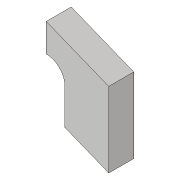
# Autodesk Inventor part: At Angle Linear Dim
Saved by Autodesk Inventor 2018.3 (Build 223284000, 284)
## iProperties
Created: 2020-03-26
Part Number: At Angle Linear Dim
Material: Generic
Document SubType Name: Modeling
Designer: MattBussey
Density: 1 g/cm^3
Appearance: Default
RuleStatus: InUse
Author: MattBussey
Autodesk Inventor part; units mm, degrees
ref_plane "YZ Plane" through (0, 0, 0) normal (1, 0, 0) x (0, 1, 0)
ref_plane "XZ Plane" through (0, 0, 0) normal (0, 1, 0) x (-1, 0, 0)
ref_plane "XY Plane" through (0, 0, 0) normal (0, 0, 1) x (1, 0, 0)
sketch "Sketch1" plane through (0, 0, 0) normal (0, 0, 1) x (1, 0, 0)
  line L0 (0, 0) -> (-63.5, 25.4)
  line L1 (-63.5, 25.4) -> (-63.5, 76.2)
  line L2 (-63.5, 76.2) -> (0, 76.2)
  line L3 (0, 76.2) -> (0, 0)
  line L4 (-63.5, 76.2) -> (-63.5, 101.6)
  line L5 (-63.5, 101.6) -> (0, 76.2)
  line L6 (0, 76.2) -> (0, 101.6) construction
  dimension "d0" = 76.2
  dimension "d13" = 25.4
  dimension "bottomAngle" = 68.199
  dimension "d16" = 25.4
  dimension "d17" = 68.199
  dimension "d18" = 21.801
  dimension "d19" = 63.5
  constraints: 14 end point, 3 vertical, 1 horizontal, 1 parallel
  measures "d0" distance of L2.end L0.start
  measures "d13" distance of L1.end L4.end
  measures "bottomAngle" angle of L0 L3
  measures "d16" distance of L2.end L6.end
  measures "d17" angle of L5 L6
  measures "d18" angle of L2 L5
  measures "d19" distance between parallel lines of L3 L1
extrude "Extrusion1" add sketch "Sketch1" along normal blind 25.4
sketch "Sketch2" plane through (0, 0, 25.4) normal (0, 0, 1) x (1, 0, 0)
  line L0 (-63.5, 0) -> (-44.45, 0)
  line L1 (-44.45, 0) -> (-44.45, 73.025)
  line L2 (-44.45, 73.025) -> (-63.5, 73.025)
  line L3 (-63.5, 73.025) -> (-63.5, 0)
  line L4 (-63.5, 101.6) -> (-63.5, 25.4) projected
  point P0 (0, 0)
  dimension "d7" = 19.05
  dimension "d8" = 73.025
  constraints: 8 end point, 2 parallel, 1 collinear, 1 horizontal, 1 perpendicular, 1 point on line
  measures "d7" distance of L0.start L0.end
  measures "d8" distance of L0.end L1.end
extrude "Extrusion2" cut sketch "Sketch2" against normal through all
fillet "Fillet1" radius 19.05 1 edges at (-44.45, 73.025, 12.7)
sketch "Sketch3" plane through (0, 0, 25.4) normal (0, 0, 1) x (1, 0, 0)
  line L0 (-44.45, 0) -> (-3.175, 0) projected
  line L1 (-44.45, 53.975) -> (-44.45, 17.78) projected
  line L2 (0, 76.2) -> (-63.5, 101.6) projected
  line L3 (-3.175, 0) -> (-44.45, 16.51)
  constraints: 2 end point, 1 parallel, 1 point on line
body "Solid1"
